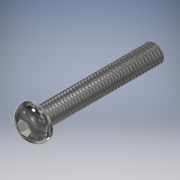
# Autodesk Inventor part: вал м8 на 400мм
Saved by Autodesk Inventor 2017 (Build 210142000, 142)
## iProperties
Part Number: вал м8 на 400мм
Material: Типовые
Document SubType Name: Modeling
Designer: alcapone
Density: 1 g/cm^3
Appearance: Сталь — полированная
Author: alcapone
Autodesk Inventor part; units mm, degrees
ref_plane "YZ Plane" through (0, 0, 0) normal (1, 0, 0) x (0, 1, 0)
ref_plane "XZ Plane" through (0, 0, 0) normal (0, 1, 0) x (-1, 0, 0)
ref_plane "XY Plane" through (0, 0, 0) normal (0, 0, 1) x (1, 0, 0)
sketch "Эскиз1" plane through (0, 0, 0) normal (0, 1, 0) x (-1, 0, 0)
  circle A0 centre (0, 0) radius 1.5
  line L0 (-1.1547, 0) -> (-0.5774, 1)
  line L1 (-0.5774, 1) -> (0.5774, 1)
  line L2 (0.5774, 1) -> (1.1547, 0)
  line L3 (1.1547, 0) -> (0.5774, -1)
  line L4 (0.5774, -1) -> (-0.5774, -1)
  line L5 (-0.5774, -1) -> (-1.1547, 0)
  circle A1 centre (0, 0) radius 2.75
  dimension "d0" = 3
  dimension "d17" = 2
  dimension "d33" = 5.5
  constraints: 12 end point, 3 coincident, 2 centre point, 13 other
  measures "d0" diameter of A0
  measures "d17" distance between parallel lines of L1 L4
  measures "d33" diameter of A1
extrude "Выдавливание1" add sketch "Эскиз1" along normal blind 15 contours A0 | L0 L1 L2 L3 L4 L5
extrude "Выдавливание3" add sketch "Эскиз1" against normal blind 2 contours A0 | A1
fillet "Сопряжение1" radius 1.72 1 edges at (2.75, -2, 0)
extrude "Выдавливание4" add sketch "Эскиз1" against normal blind 0.5 contours L0 L1 L2 L3 L4 L5
chamfer "Фаска1" distance 0.5 angle 45 1 edges at (1.5, 15, 0)
thread "Резьба4" size "M3x0.5" class "6g" standard "ANSI Metric M Profile" full length
sketch "Эскиз14" plane through (0, 14.5, 0) normal (1, 0, 0) x (0, 0, 1)
  line L0 (1.5, 0) -> (1.5, 14.5)
  line L1 (1.5, 14.5) -> (1.2294, 14.5)
  line L2 (1.2294, 14.5) -> (1.2294, 0)
  line L3 (1.2294, 0) -> (1.5, 0)
  line L4 (0, -3.9377) -> (0, 19.9075) projected
  constraints: 8 end point
revolve "Вращение8" cut sketch "Эскиз14" angle 360 about axis through (0, 14.5, 0) along (0, -1, 0)
sketch "Эскиз15" plane through (0, 14.5, 0) normal (1, 0, 0) x (0, 0, 1)
  line L0 (1.5, 0) -> (1.5, 14.5)
  line L1 (1.5, 14.5) -> (1.2294, 14.5)
  line L2 (1.2294, 14.5) -> (1.2294, 0)
  line L3 (1.2294, 0) -> (1.5, 0)
  line L4 (0, -3.9377) -> (0, 19.9075) projected
  constraints: 8 end point
revolve "Вращение9" add sketch "Эскиз15" angle 360 about axis through (0, 14.5, 0) along (0, -1, 0) separate body
sketch "Эскиз13" plane through (0, 14.5, 0) normal (-1, 0, 0) x (0, -1, 0)
  line L0 (-0.25, -1.1211) -> (-0.3305, -1.2606) construction
  line L1 (-0.25, -1.1211) -> (-0.1695, -1.2606) construction
  line L2 (-0.25, -1.1211) -> (-0.25, -1.2294) construction
  line L3 (-0.3125, -1.2294) -> (-0.2764, -1.2294) construction
  line L4 (0, -1.5541) -> (0.0312, -1.5) construction
  line L5 (-0.5, -1.5541) -> (-0.5312, -1.5) construction
  line L6 (-0.5312, -1.5) -> (-0.5, -1.5) construction
  line L7 (-0.4688, -1.5) -> (-0.5, -1.5541) construction
  arc A0 (-0.2764, -1.2294) -> (-0.3305, -1.2606) centre (-0.2764, -1.2919) ccw
  arc A1 (-0.1695, -1.2606) -> (-0.2236, -1.2294) centre (-0.2236, -1.2919) ccw
  line L8 (0, -1.5541) -> (0, -1.5) construction
  line L9 (-0.5, -1.5541) -> (-0.5, -1.5) construction
  arc A2 (-0.0403, -1.4844) -> (-0.0132, -1.5) centre (-0.0132, -1.4688) ccw
  line L10 (-0.1695, -1.2606) -> (-0.0403, -1.4844)
  line L11 (-0.2764, -1.2294) -> (-0.2236, -1.2294)
  line L12 (-0.3305, -1.2606) -> (-0.4597, -1.4844)
  line L13 (-0.0132, -1.5) -> (0, -1.5) construction
  line L14 (0, -1.5) -> (0.0312, -1.5) construction
  arc A3 (-0.4868, -1.5) -> (-0.4597, -1.4844) centre (-0.4868, -1.4688) ccw
  line L15 (-0.4597, -1.4844) -> (-0.4688, -1.5) construction
  line L16 (-0.5, -1.5) -> (-0.4868, -1.5) construction
  line L17 (-0.4868, -1.5) -> (-0.0132, -1.5)
  line L18 (0, 0) -> (0.4413, 0)
  line L19 (0, 0) -> (0, 0.419)
  line L20 (0, -1.5541) -> (-0.0403, -1.4844) construction
  dimension "d113" = 0.1082
  dimension "d114" = 0.0625
  dimension "d115" = 0.0312
  dimension "d116" = 0.0541
  dimension "d117" = 0.5
  dimension "Эскиз13_MajorRadius" = 1.5
  dimension "d119" = 60
  dimension "Эскиз13_ThreadOffset" = 0
  dimension "Эскиз13_MinorRadius" = 1.2294
  constraints: 42 end point, 17 tangent, 8 point on circle, 6 parallel, 5 collinear, 4 centre point, 3 point on line, 3 vertical, 2 equal radius, 2 horizontal, 2 perpendicular, 1 equal length, 1 midpoint, 4 other
  measures "d113" distance from line of L0.start L3
  measures "d114" radius of A0
  measures "d115" radius of A2
  measures "d116" distance from line of L14 L4.start
  measures "d117" distance between parallel lines of L8 L9
  measures "Эскиз13_MajorRadius" distance between parallel lines of L14 L18
  measures "d119" angle of L10 L12
  measures "Эскиз13_ThreadOffset" distance between parallel lines of L19 L8
  measures "Эскиз13_MinorRadius" distance between parallel lines of L18 L11
coil "Пружина6" sketch "Эскиз13" operation cut axis through (0, 14.5, 0) along (0, -1, 0) pitch 0.5005 turns 30.969031 hand right bodies 2
equation "\"d113\" = 0.216506 * Эскиз13_Pitch"
equation "\"d114\" = d122"
equation "\"d115\" = 0.0625 * Эскиз13_Pitch"
equation "\"d116\" = 0.108253 * Эскиз13_Pitch"
equation "\"d117\" = Эскиз13_Pitch"
equation "\"d119\" = d124"
equation "\"d51\" = 55deg"
equation "\"Эскиз4_Pitch\" = 0.8"
equation "\"d74\" = 0.125 * Эскиз7_Pitch"
equation "\"Эскиз7_Pitch\" = 0.8"
equation "\"d76\" = 60deg"
equation "\"d98\" = 0.125 * Эскиз10_Pitch"
equation "\"Эскиз10_Pitch\" = 0.5"
equation "\"d100\" = 60deg"
equation "\"d122\" = 0.125 * Эскиз13_Pitch"
equation "\"Эскиз13_Pitch\" = 0.5"
equation "\"d124\" = 60deg"
